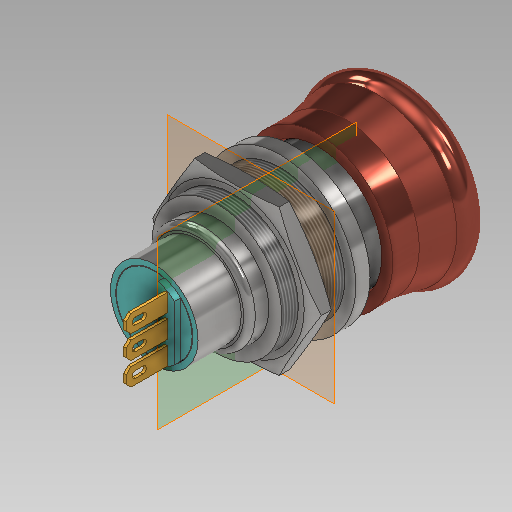
# Autodesk Inventor part: E-Stop
Saved by Autodesk Inventor 2020 (Build 240168000, 168)
## iProperties
Created: 2022-03-29
Part Number: E-Stop
Material: Stainless Steel
Document SubType Name: Modeling
Designer: Suriyan.S
Density: 8 g/cm^3
Appearance: Silver
Author: Suriyan.S
Autodesk Inventor part; units mm, degrees
ref_plane "YZ Plane" through (0, 0, 0) normal (1, 0, 0) x (0, 1, 0)
ref_plane "XZ Plane" through (0, 0, 0) normal (0, 1, 0) x (-1, 0, 0)
ref_plane "XY Plane" through (0, 0, 0) normal (0, 0, 1) x (1, 0, 0)
sketch "Sketch1" plane through (0, 0, 0) normal (0, 0, 1) x (1, 0, 0)
  circle A0 centre (0, 0) radius 12.89
  dimension "d0" = 25.78
  constraints: 1 centre point, 1 coincident
  measures "d0" diameter of A0
extrude "Extrusion1" add sketch "Sketch1" against normal blind 2.4
sketch "Sketch2" plane through (0, 0, -2.4) normal (0, 0, -1) x (-1, 0, 0)
  circle A0 centre (0, 0) radius 12.89 construction
  circle A1 centre (0, 0) radius 10.285
  dimension "d3" = 20.57
  constraints: 1 centre point, 1 coincident
  measures "d3" diameter of A1
extrude "Extrusion2" add sketch "Sketch2" along normal blind 6
sketch "Sketch3" plane through (0, 0, 0) normal (0, 0, 1) x (1, 0, 0)
  circle A0 centre (0, 0) radius 12.89 construction
  circle A1 centre (0, 0) radius 11
  dimension "d6" = 22
  constraints: 1 centre point, 1 coincident
  measures "d6" diameter of A1
extrude "Extrusion3" add sketch "Sketch3" along normal blind 10.7
sketch "Sketch4" plane through (0, 0, 10.7) normal (0, 0, 1) x (1, 0, 0)
  circle A0 centre (0, 0) radius 11 construction
  circle A1 centre (0, 0) radius 8.815
  dimension "d9" = 17.63
  constraints: 1 centre point, 1 coincident
  measures "d9" diameter of A1
extrude "Extrusion4" add sketch "Sketch4" along normal blind 3.3
sketch "Sketch5" plane through (0, 0, 14) normal (0, 0, 1) x (1, 0, 0)
  circle A0 centre (0, 0) radius 8.815 construction
  circle A1 centre (0, 0) radius 7.425
  dimension "d12" = 14.85
  constraints: 1 centre point
  measures "d12" diameter of A1
extrude "Extrusion5" add sketch "Sketch5" along normal blind 7.34
sketch "Sketch6" plane through (0, 0, 21.34) normal (0, 0, 1) x (1, 0, 0)
  circle A0 centre (0, 0) radius 7.425 projected
  line L0 (1.625, -16.212) -> (4.425, -16.212)
  line L1 (4.425, -16.212) -> (4.425, 19.0425)
  line L2 (4.425, 19.0425) -> (1.625, 19.0425)
  line L3 (1.625, 19.0425) -> (1.625, -16.212)
  point P0 (1.625, 7.245)
  point P1 (1.625, -7.245)
  point P2 (4.425, -5.9624)
  point P3 (4.425, 5.9624)
  dimension "d15" = 5.8
  dimension "d16" = 2.8
  constraints: 8 end point, 2 parallel, 1 horizontal, 1 perpendicular
  measures "d15" distance edge to line of A0 L3
  measures "d16" distance between parallel lines of L3 L1
extrude "Extrusion6" add sketch "Sketch6" along normal blind 1 contours L1 A0 L3
sketch "Sketch7" plane through (0, 0, 21.34) normal (0, 0, 1) x (1, 0, 0)
  arc A0 (1.625, 7.245) -> (1.625, -7.245) centre (0, 0) ccw construction
  circle A1 centre (0, 0) radius 7.425
  circle A2 centre (0, 0) radius 6.425
  dimension "d19" = 1
  constraints: 2 centre point, 2 coincident, 1 concentric
  measures "d19" radial gap between concentric circles of A0 A2
extrude "Extrusion7" cut sketch "Sketch7" along normal through all
ref_plane "Work Plane1" through (3.025, -6.2161, 21.34) normal (-1, 0, 0) x (0, 0, 1)
sketch "Sketch8" plane through (3.025, -6.2161, 21.34) normal (-1, 0, 0) x (0, 0, 1)
  line L0 (1, 12.4322) -> (1, 0) projected
  line L1 (1, 0.8) -> (8, 0.8)
  line L2 (8, 0.8) -> (8, 3.8)
  line L3 (8, 3.8) -> (1, 3.8)
  line L4 (0.9658, 11.6322) -> (8, 11.6322)
  line L5 (8, 11.6322) -> (8, 8.6322)
  line L6 (8, 8.6322) -> (0.9658, 8.6322)
  line L7 (0.9658, 8.6322) -> (0.9658, 11.6322)
  line L8 (1, 4.7161) -> (8, 4.7161)
  line L9 (8, 4.7161) -> (8, 7.7161)
  line L10 (8, 7.7161) -> (1, 7.7161)
  line L11 (1, 7.7161) -> (1, 4.7161)
  line L12 (-7.34, -2.5989) -> (-7.34, 15.0311) construction
  line L13 (6.42, 2.3) -> (5.18, 2.3) construction
  line L14 (6.42, 2.88) -> (5.18, 2.88)
  line L15 (5.18, 1.72) -> (6.42, 1.72)
  arc A0 (6.42, 1.72) -> (6.42, 2.88) centre (6.42, 2.3) ccw
  arc A1 (5.18, 2.88) -> (5.18, 1.72) centre (5.18, 2.3) ccw
  line L16 (6.42, 6.2161) -> (5.18, 6.2161) construction
  line L17 (6.42, 5.6361) -> (5.18, 5.6361)
  line L18 (5.18, 6.7961) -> (6.42, 6.7961)
  arc A2 (6.42, 5.6361) -> (6.42, 6.7961) centre (6.42, 6.2161) ccw
  arc A3 (5.18, 6.7961) -> (5.18, 5.6361) centre (5.18, 6.2161) ccw
  line L19 (6.42, 10.1322) -> (5.18, 10.1322) construction
  line L20 (6.42, 9.5522) -> (5.18, 9.5522)
  line L21 (5.18, 10.7122) -> (6.42, 10.7122)
  arc A4 (6.42, 9.5522) -> (6.42, 10.7122) centre (6.42, 10.1322) ccw
  arc A5 (5.18, 10.7122) -> (5.18, 9.5522) centre (5.18, 10.1322) ccw
  line L22 (0, 0) -> (1, 0) construction
  line L23 (1, 12.4322) -> (0, 12.4322) construction
  point P0 (-21.34, 6.2161)
  point P1 (-7.34, 6.2161)
  point P2 (8, 6.2161)
  point P3 (5.8, 2.3)
  point P4 (5.8, 6.2161)
  point P5 (5.8, 10.1322)
  point P6 (8, 10.1322)
  point P7 (8, 2.3)
  point P8 (4.6, 2.3)
  point P9 (7, 2.3)
  point P10 (1, 11.6322)
  point P11 (1, 8.6322)
  point P12 (1, 0.8)
  dimension "d22" = 3
  dimension "d23" = 7
  dimension "d25" = 4.8
  dimension "d26" = 1.16
  dimension "d27" = 2.4
  dimension "d28" = 0.8
  dimension "d29" = 0.8
  constraints: 47 end point, 14 point on circle, 12 tangent, 10 parallel, 7 midpoint, 6 centre point, 5 point on line, 4 equal length, 4 horizontal, 4 horizontal alignment, 3 perpendicular, 2 equal radius, 2 vertical alignment, 1 other
  measures "d22" distance of L8.end L9.end
  measures "d23" distance of L1.start L1.end
  measures "d25" distance from line of L0 point (5.8, 6.216)
  measures "d26" distance between parallel lines of L14 L15
  measures "d27" distance of point (7, 2.3) point (4.6, 2.3)
  measures "d28" distance between parallel lines of L1 L22
extrude "Extrusion8" add sketch "Sketch8" along normal mid plane 0.45 separate body contours L10 L9 L8 L0 | L0 L4 L5 L6 | L3 L2 L1 L0
chamfer "Chamfer1" distance 0.8 angle 45 6 edges at (3.025, -5.4161, 29.34) (3.025, -2.4161, 29.34) (3.025, -1.5, 29.34) (3.025, 1.5, 29.34) (3.025, 2.4161, 29.34) (3.025, 5.4161, 29.34)
sketch "Sketch10" plane through (0, 0, 0) normal (0, 1, 0) x (-1, 0, 0)
  line L0 (-12.89, -2.4) -> (12.89, -2.4) construction
  line L1 (14.5, -21.2) -> (-14.5, -21.2)
  line L2 (-14.5, -21.2) -> (-14.5, -6.5)
  line L3 (-14.5, -6.5) -> (14.5, -6.5)
  line L4 (14.5, -6.5) -> (14.5, -21.2)
  line L5 (14.5, -21.2) -> (-14.5, -6.5) construction
  line L6 (-14.5, -21.2) -> (14.5, -6.5) construction
  line L7 (-12.65, -6.5) -> (12.65, -6.5)
  line L8 (12.65, -6.5) -> (12.65, -11)
  line L9 (12.65, -11) -> (-12.65, -11)
  line L10 (-12.65, -11) -> (-12.65, -6.5)
  line L11 (-11.65, -21.2) -> (11.65, -21.2)
  line L12 (11.65, -21.2) -> (11.65, -32.8003)
  line L13 (11.65, -32.8003) -> (-11.65, -32.8003) construction
  line L14 (-11.65, -32.8003) -> (-11.65, -21.2)
  circle A0 centre (-11.65, -18.35) radius 2.85
  line L15 (-12.65, -11) -> (-13.67, -16.3395)
  line L16 (-10.785, -6.5) -> (-10.785, -11)
  line L17 (-10.285, -2.4) -> (-10.285, -8.4) construction
  line L18 (0, -6.5) -> (0, -32.8003)
  line L19 (-10.285, -8.4) -> (10.285, -8.4) construction
  point P0 (0, 0)
  point P1 (0, -13.85)
  point P2 (0, -13.85)
  point P3 (0, -11)
  point P4 (0, -13.85)
  point P5 (0, -21.2)
  point P6 (0, -21.2)
  point P7 (0, -11)
  dimension "d35" = 29
  dimension "d36" = 4.1
  dimension "d37" = 14.7
  dimension "d38" = 4.5
  dimension "d39" = 25.3
  dimension "d40" = 23.3
  dimension "d41" = 13.67
  dimension "d42" = 0.5
  constraints: 34 end point, 8 midpoint, 6 parallel, 5 perpendicular, 4 point on line, 3 horizontal, 3 vertical alignment, 2 point on circle, 2 tangent, 1 centre point
  measures "d35" distance of L1.start L1.end
  measures "d36" distance between parallel lines of L0 L3
  measures "d37" distance of L1.end L2.end
  measures "d38" distance of L9.end L7.start
  measures "d39" distance of L8.end L9.end
  measures "d40" distance of L12.end L13.end
  measures "d41" horizontal distance of point (0, -21.2) L15.end
  measures "d42" distance between parallel lines of L16 L17
revolve "Revolution1" add sketch "Sketch10" angle 360 about axis through (0, 0, -6.5) along (0, 0, -1) separate body contours L1 A0 L15 L9 L18 | A0 | L9 L10 L3 L16
thread "Thread1" size "M22x0.5" class "6g" standard "ANSI Metric M Profile" full length
fillet "Fillet1" radius 1 1 edges at (-8.815, 0, 14)
sketch "Sketch11" plane through (0, 0, 21.34) normal (0, 0, 1) x (1, 0, 0)
  circle A0 centre (0, 0) radius 7.425 construction
  circle A1 centre (0, 0) radius 6.425
  circle A2 centre (0, 0) radius 6.525
  dimension "d47" = 1
  dimension "d48" = 0.1
  constraints: 2 centre point
  measures "d47" radial gap between concentric circles of A0 A1
  measures "d48" radial gap between concentric circles of A1 A2
extrude "Extrusion9" cut sketch "Sketch11" against normal blind 1 bodies 1
sketch "Sketch12" plane through (0, 0, -21.2) normal (0, 0, -1) x (-1, 0, 0)
  circle A0 centre (0, 0) radius 11.65 construction
  circle A1 centre (0, 0) radius 9.5
  circle A2 centre (0, 0) radius 8
  line L0 (0, 0) -> (-9.5, 0)
  line L1 (0, 0) -> (4.75, -8.2272)
  line L2 (0, 0) -> (4.75, 8.2272)
  line L3 (0, 0) -> (-8.2272, -4.75)
  line L4 (0, 0) -> (-8.2272, 4.75)
  line L5 (-8.2272, 4.75) -> (-8.8768, 5.125)
  line L6 (-8.8768, 5.125) -> (-6.3863, 5.9814)
  line L7 (-6.2787, 3.625) -> (-6.3863, 5.9814)
  circle A3 centre (0, 0) radius 8.75 construction
  point P0 (-7.5777, 4.375)
  point P1 (-6.9282, -4)
  point P2 (-6.9282, 4)
  dimension "d51" = 1.5
  dimension "d52" = 16
  dimension "d53" = 120
  dimension "d54" = 120
  dimension "d55" = 30
  dimension "d56" = 30
  dimension "d57" = 3
  dimension "d58" = 1.5
  dimension "d59" = 2
  dimension "d60" = 0.75
  constraints: 16 end point, 7 point on circle, 3 centre point, 3 coincident, 2 point on line, 1 collinear, 1 horizontal
  measures "d51" radial gap between concentric circles of A2 A1
  measures "d52" diameter of A2
  measures "d53" angle of L2 L0
  measures "d54" angle of L1 L0
  measures "d55" angle of L4 L0
  measures "d56" angle of L0 L3
  measures "d57" distance of L7.start L5.end
  measures "d58" distance of L7.start A3.start
  measures "d59" distance of A3.start L6.end
  measures "d60" radial gap between concentric circles of A3 A2
extrude "Extrusion10" add sketch "Sketch12" along normal blind 0.001 separate body contours L6 L7 A2 L4 A1 | A1 L5 L6 | A1 L0 A2 L3 | L4 A2 L0 A1 | L7 L4 A2
pattern_circular "Circular Pattern1" count 3 over 360 about axis through (0, 0, -8.75) along (0, 0, 1) of "Extrusion10" bodies 4
ref_plane "Work Plane2" through (0, 0, 5) normal (0, 0, 1) x (1, 0, 0)
sketch "Sketch13" plane through (0, 0, 5) normal (0, 0, 1) x (1, 0, 0)
  circle A0 centre (0, 0) radius 12.89 construction
  line L0 (-14.3183, 0) -> (-7.1591, 12.4)
  line L1 (-7.1591, 12.4) -> (7.1591, 12.4)
  line L2 (7.1591, 12.4) -> (14.3183, 0)
  line L3 (14.3183, 0) -> (7.1591, -12.4)
  line L4 (7.1591, -12.4) -> (-7.1591, -12.4)
  line L5 (-7.1591, -12.4) -> (-14.3183, 0)
  circle A1 centre (0, 0) radius 11 projected
  dimension "d67" = 24.8
  constraints: 12 end point, 1 coincident, 1 horizontal alignment, 13 other
  measures "d67" distance between parallel lines of L2 L5
extrude "Extrusion11" add sketch "Sketch13" along normal blind 2.9 separate body
sketch "Sketch14" plane through (0, 0, 0) normal (1, 0, 0) x (0, 1, 0)
  line L0 (-12.4, 7.9) -> (0, 7.9) construction
  line L1 (-12, 7.9) -> (-15, 7.1)
  line L2 (-12.4, 5.0222) -> (-12.4, 7.9) construction
  line L3 (-12.4, 7.9) -> (-12, 7.9)
  line L4 (-12.7962, 5) -> (0, 5) construction
  line L5 (-15, 5) -> (-12, 5)
  line L6 (-15, 5.8) -> (-12, 5)
  line L7 (-15, 5) -> (-15, 5.8)
  line L8 (0, -4.339) -> (0, 11.9739)
  line L9 (-11, 7.9) -> (-11, 5) construction
  line L10 (-11, 7.9) -> (-11, 5) construction
  line L11 (0, 7.9) -> (-12.4, 7.9) construction
  line L12 (0, 5) -> (-12.4, 5) construction
  line L13 (-15, 7.1) -> (-15, 7.9)
  line L14 (-15, 7.9) -> (-12, 7.9)
  point P0 (0, 0)
  point P1 (-12.7962, 5.0222)
  dimension "d70" = 0.8
  dimension "d71" = 0.8
  dimension "d72" = 3
  dimension "d73" = 3
  dimension "d74" = 1
  constraints: 16 end point, 2 horizontal, 2 vertical, 1 collinear, 1 perpendicular, 1 point on line, 1 vertical alignment, 3 other
  measures "d71" distance from line of L1.end L0
  measures "d72" horizontal distance of L1.start L1.end
  measures "d73" horizontal distance of L6.start L5.end
  measures "d74" distance from line of L9 L1.start
revolve "Revolution2" cut sketch "Sketch14" angle 360 about axis through (0, 0, -4.339) along (0, 0, 1) bodies 5
equation "\"d29\" = d28"
equation "\"d54\" = d53"
equation "\"d56\" = d55"
equation "\"d58\" = 0.5 * d57"
equation "\"d71\" = d70"
equation "\"d73\" = d72"
body "Solid1"
body "Solid2"
body "Solid3"
body "Solid4"
body "Solid5"
